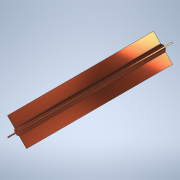
# Autodesk Inventor part: propeller
Saved by Autodesk Inventor 2020 (Build 240168000, 168)
## iProperties
Created: 2020-04-30
Part Number: propeller
Material: Generic
Document SubType Name: Modeling
Designer: LENOVO
Density: 1 g/cm^3
Appearance: Default
Author: LENOVO
Autodesk Inventor part; units mm, degrees
ref_plane "YZ Plane" through (0, 0, 0) normal (1, 0, 0) x (0, 1, 0)
ref_plane "XZ Plane" through (0, 0, 0) normal (0, 1, 0) x (-1, 0, 0)
ref_plane "XY Plane" through (0, 0, 0) normal (0, 0, 1) x (1, 0, 0)
sketch "Sketch1" plane through (0, 0, 0) normal (0, 0, 1) x (1, 0, 0)
  arc A0 (-1, 2.2913) -> (1, 2.2913) centre (0, 0) ccw
  line L0 (33.5703, 31.449) -> (9.177, 7.0557)
  line L1 (31.449, 33.5703) -> (7.0557, 9.177)
  line L2 (-33.5703, 31.449) -> (-9.177, 7.0557)
  line L3 (-31.449, 33.5703) -> (-7.0557, 9.177)
  line L4 (33.5703, -31.449) -> (9.177, -7.0557)
  line L5 (31.449, -33.5703) -> (7.0557, -9.177)
  line L6 (-33.5703, -31.449) -> (-9.177, -7.0557)
  line L7 (-31.449, -33.5703) -> (-7.0557, -9.177)
  arc A1 (-31.449, 33.5703) -> (-33.5703, 31.449) centre (0, 0) ccw
  arc A2 (33.5703, 31.449) -> (31.449, 33.5703) centre (0, 0) ccw
  arc A3 (-33.5703, -31.449) -> (-31.449, -33.5703) centre (0, 0) ccw
  arc A4 (31.449, -33.5703) -> (33.5703, -31.449) centre (0, 0) ccw
  arc A5 (-8.826, 4.7012) -> (-8.826, -4.7012) centre (0, 0) ccw
  arc A6 (-4.7012, -8.826) -> (4.7012, -8.826) centre (0, 0) ccw
  arc A7 (8.826, -4.7012) -> (8.826, 4.7012) centre (0, 0) ccw
  arc A8 (4.7012, 8.826) -> (-4.7012, 8.826) centre (0, 0) ccw
  arc A9 (-8.826, 4.7012) -> (-9.177, 7.0557) centre (-10.5912, 5.6415) ccw
  arc A10 (-9.177, -7.0557) -> (-8.826, -4.7012) centre (-10.5912, -5.6415) ccw
  arc A11 (-4.7012, -8.826) -> (-7.0557, -9.177) centre (-5.6415, -10.5912) ccw
  arc A12 (7.0557, -9.177) -> (4.7012, -8.826) centre (5.6415, -10.5912) ccw
  arc A13 (8.826, -4.7012) -> (9.177, -7.0557) centre (10.5912, -5.6415) ccw
  arc A14 (9.177, 7.0557) -> (8.826, 4.7012) centre (10.5912, 5.6415) ccw
  arc A15 (4.7012, 8.826) -> (7.0557, 9.177) centre (5.6415, 10.5912) ccw
  arc A16 (-7.0557, 9.177) -> (-4.7012, 8.826) centre (-5.6415, 10.5912) ccw
  line L8 (-1, 5.5) -> (1, 5.5)
  line L9 (1, 5.5) -> (1, 2.2913)
  line L10 (-1, 2.2913) -> (-1, 5.5)
  line L11 (-1, 5.5) -> (1, 2.5) construction
  line L12 (1, 5.5) -> (-1, 2.5) construction
  point P0 (8.0517, 5.9304)
  point P1 (5.9304, 8.0517)
  point P2 (-8.0517, 5.9304)
  point P3 (-5.9304, 8.0517)
  point P4 (8.0517, -5.9304)
  point P5 (5.9304, -8.0517)
  point P6 (-8.0517, -5.9304)
  point P7 (-5.9304, -8.0517)
  point P8 (0, 4)
  dimension "d0" = 5
  dimension "d10" = 2
  dimension "d18" = 46
  dimension "d19" = 46
  dimension "d20" = 46
  dimension "d21" = 46
  constraints: 42 point on circle, 26 end point, 17 centre point, 16 tangent, 10 point on line, 7 equal radius, 2 coincident, 2 midpoint, 1 horizontal, 1 parallel, 1 perpendicular
  measures "d0" diameter of A0
  measures "d10" radius of A9
  measures "d18" radius of A1
  measures "d19" radius of A2
  measures "d20" radius of A3
  measures "d21" radius of A4
extrude "Extrusion2" add sketch "Sketch1" against normal blind 494
body "Solid2"
